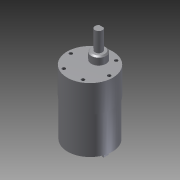
# Autodesk Inventor part: Motor12V
Saved by Autodesk Inventor 2011 SP2 (Build 150309200, 309)
## iProperties
Created: 2015-10-13
Part Number: Motor12V
Document SubType Name: Modeling
Designer: Ernest
Density: 1 g/cm^3
Mass: 54.1047 g
Surface Area: 93.1269 cm^2
Volume: 54.1047 cm^3
Author: Ernest
Autodesk Inventor part; units mm, degrees
ref_plane "YZ Plane" through (0, 0, 0) normal (1, 0, 0) x (0, 1, 0)
ref_plane "XZ Plane" through (0, 0, 0) normal (0, 1, 0) x (-1, 0, 0)
ref_plane "XY Plane" through (0, 0, 0) normal (0, 0, 1) x (1, 0, 0)
sketch "Sketch1" plane through (0, 0, 0) normal (0, 0, 1) x (1, 0, 0)
  circle A0 centre (0, 0) radius 18.4
  dimension "d0" = 36.8
  constraints: 1 centre point, 1 coincident
  measures "d0" diameter of A0
extrude "Extrusion1" add sketch "Sketch1" along normal blind 22
sketch "Sketch2" plane through (0, 0, 0) normal (0, 0, -1) x (-1, 0, 0)
  circle A0 centre (0, 0) radius 18.4 projected
  circle A1 centre (0, 0) radius 18
  dimension "d3" = 36
  constraints: 1 centre point, 1 coincident
  measures "d3" diameter of A1
extrude "Extrusion2" add sketch "Sketch2" along normal blind 30 contours A1
sketch "Sketch3" plane through (0, 0, -30) normal (0, 0, -1) x (-1, 0, 0)
  circle A0 centre (0, 0) radius 18 projected
  circle A1 centre (0, 0) radius 17.75
  circle A2 centre (0, 0) radius 5
  line L0 (-12, -2) -> (-13, -2)
  line L1 (-13, -2) -> (-13, 2)
  line L2 (-13, 2) -> (-12, 2)
  line L3 (-12, 2) -> (-12, -2)
  line L4 (12, 2) -> (13, 2)
  line L5 (13, 2) -> (13, -2)
  line L6 (13, -2) -> (12, -2)
  line L7 (12, -2) -> (12, 2)
  dimension "d6" = 35.5
  dimension "d7" = 10
  dimension "d8" = 4
  dimension "d9" = 4
  dimension "d10" = 1
  dimension "d11" = 1
  dimension "d12" = 2
  dimension "d13" = 2
  dimension "d14" = 12
  dimension "d15" = 12
  constraints: 16 end point, 4 parallel, 2 centre point, 2 coincident, 2 horizontal, 2 perpendicular
  measures "d6" diameter of A1
  measures "d7" diameter of A2
  measures "d8" distance of L0.end L1.end
  measures "d9" distance of L4.end L5.end
  measures "d10" distance of L5.end L6.end
  measures "d11" distance of L0.start L0.end
  measures "d12" distance from line of A0.centre L2
  measures "d13" distance from line of A0.centre L4
  measures "d14" distance from line of A0.centre L7
  measures "d15" distance from line of A0.centre L3
extrude "Extrusion3" add sketch "Sketch3" along normal blind 5.6 contours L0 L1 L2 L3 | L4 L5 L6 L7
extrude "Extrusion4" add sketch "Sketch3" along normal blind 2 contours A2
extrude "Extrusion5" cut sketch "Sketch3" against normal blind 1 contours A1
sketch "Sketch4" plane through (0, 0, 22) normal (0, 0, 1) x (1, 0, 0)
  circle A0 centre (0, 0) radius 18.4 projected
  circle A1 centre (0, 7) radius 6
  line L0 (15.5, 0) -> (0, 0) construction
  line L1 (12, 2) -> (12, -2) construction
  dimension "d22" = 7
  dimension "d23" = 12
  dimension "d28" = 15.5
  constraints: 2 end point, 1 centre point, 1 perpendicular
  measures "d22" distance of L0.end A1.centre
  measures "d23" diameter of A1
  measures "d28" distance of L0.start L0.end
extrude "Extrusion6" add sketch "Sketch4" along normal blind 6.5 contours A1
hole "Hole1" at (15.5, 0, 22) direction (0, 0, -1) diameter 2.621 depth 8 tip angle 118 thread size "M3x0.35" class "6H" standard "ANSI Metric M Profile"
pattern_circular "Circular Pattern1" count 6 over 360 about axis through (0, 0, 0) along (0, 0, 1) of "Hole1"
chamfer "Chamfer1" distance 1 angle 45 1 edges at (-6, 7, 28.5)
sketch "Sketch5" plane through (0, 7, 28.5) normal (0, 0, 1) x (1, 0, 0)
  circle A0 centre (0, 0) radius 5 projected
  circle A1 centre (0, 0) radius 3
  point P0 (0, -7)
  dimension "d42" = 6
  constraints: 1 centre point, 1 coincident
  measures "d42" diameter of A1
extrude "Extrusion7" add sketch "Sketch5" along normal blind 15.5 contours A1
sketch "Sketch6" plane through (0, 7, 44) normal (0, 0, 1) x (1, 0, 0)
  circle A0 centre (0, 0) radius 3 projected
  line L0 (-1.8, 2.4) -> (1.8, 2.4)
  point P0 (0, -7)
  dimension "d45" = 5.4
  constraints: 2 end point, 2 point on circle, 1 horizontal
extrude "Extrusion8" cut sketch "Sketch6" against normal blind 12 contours L0 A0 picked at (0, 2.6)
body "Solid1"
